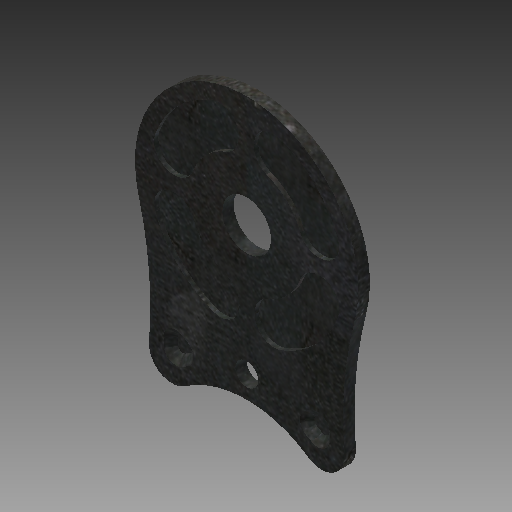
# Autodesk Inventor part: 201-09
Saved by Autodesk Inventor 2019 (Build 230136000, 136)
## iProperties
Company: Autodesk Inc.
Created: 2007-11-01
Part Number: 201-09
Document SubType Name: Modeling
Designer: Autodesk Inc.
Density: 7.85 g/cm^3
Mass: 170.342 g
Surface Area: 144.32 cm^2
Volume: 21.6997 cm^3
Material: Steel
Description: SIDE PIVOT PLATE
Appearance: Plate
Component Category: Lower Component
Author: Inventor
Autodesk Inventor part; units mm, degrees
ref_plane "YZ Plane" through (0, 0, 0) normal (1, 0, 0) x (0, 1, 0)
ref_plane "XZ Plane" through (0, 0, 0) normal (0, 1, 0) x (-1, 0, 0)
ref_plane "XY Plane" through (0, 0, 0) normal (0, 0, 1) x (1, 0, 0)
sketch "Sketch1" plane through (0, 0, 0) normal (0, 0, 1) x (1, 0, 0)
  arc A0 (37.7266, -9.8844) -> (-37.7266, -9.8844) centre (0, 0) ccw
  arc A1 (-34.0962, -52.1712) -> (-21.585, -59.437) centre (-26.125, -52.85) ccw
  arc A2 (21.585, -59.437) -> (34.0962, -52.1712) centre (26.125, -52.85) ccw
  arc A3 (-34.0962, -52.1712) -> (-37.7266, -9.8844) centre (-158.6454, -41.565) ccw
  line L0 (0, 64.9508) -> (0, -116.7047) projected
  arc A4 (21.585, -59.437) -> (-21.585, -59.437) centre (0, -90.7539) ccw
  arc A5 (37.7266, -9.8844) -> (34.0962, -52.1712) centre (158.6454, -41.565) ccw
  dimension "d0" = 16
  dimension "d2" = 78
  dimension "d3" = 52.85
  dimension "d5" = 26.125
  dimension "d8" = 317.2907
  dimension "d9" = 26.125
  dimension "d10" = 38.035
  constraints: 13 point on circle, 6 centre point, 4 tangent, 3 symmetric about line, 1 coincident, 1 point on line, 1 other
  measures "d0" diameter of A1
  measures "d2" diameter of A0
  measures "d3" vertical distance of A1.centre point (0, 0)
  measures "d5" horizontal distance of A1.centre point (0, 0)
  measures "d8" distance of A5.centre A3.centre
  measures "d9" distance from line of L0 A2.centre
  measures "d10" radius of A4
extrude "Extrusion1" add sketch "Sketch1" against normal blind 4
sketch "Sketch2" plane through (0, 0, -4) normal (0, 0, -1) x (-1, 0, 0)
  arc A0 (37.7266, -9.8844) -> (-37.7266, -9.8844) centre (0, 0) ccw projected
  arc A1 (-34.0962, -52.1712) -> (-21.585, -59.437) centre (-26.125, -52.85) ccw projected
  arc A2 (21.585, -59.437) -> (-21.585, -59.437) centre (0, -90.7539) ccw projected
  line L0 (-27.275, -50.4758) -> (-27.275, -48.2242)
  line L1 (-21.575, -51.5151) -> (-23.525, -52.6409)
  line L2 (-23.525, -46.0591) -> (-21.575, -47.1849)
  arc A3 (-23.525, -46.0591) -> (-27.275, -48.2242) centre (-24.775, -48.2242) ccw
  arc A4 (-27.275, -50.4758) -> (-23.525, -52.6409) centre (-24.775, -50.4758) ccw
  arc A5 (-21.575, -51.5151) -> (-21.575, -47.1849) centre (-22.825, -49.35) ccw
  line L3 (0, -116.7047) -> (0, 64.9508) projected
  point P0 (-27.275, 27.8761)
  point P1 (-32.4256, -57.7797)
  point P2 (-9.7764, -53.9968)
  dimension "d13" = 60
  dimension "d14" = 60
  dimension "d15" = 2.5
  dimension "d16" = 22.825
  dimension "d17" = 49.35
  dimension "d18" = 60
  dimension "d19" = 1.95
  constraints: 9 point on circle, 6 end point, 6 tangent, 3 centre point, 3 point on line, 2 equal radius
  measures "d13" angle of L1 L0
  measures "d14" angle of L1 L2
  measures "d15" radius of A3
  measures "d16" horizontal distance of A0.centre A5.centre
  measures "d17" vertical distance of A0.centre A5.centre
  measures "d18" angle of L3 L1
  measures "d19" horizontal distance of A3.centre A5.centre
extrude "Extrusion2" add sketch "Sketch2" along normal blind 2.5
chamfer "Chamfer1" distance 2.5 angle 45 6 edges at (22.55, -52.078, -4) (26.025, -52.6409, -4) (27.275, -49.35, -4) (26.025, -46.0591, -4) (22.55, -46.622, -4) (20.325, -49.35, -4)
mirror "Mirror1" about plane through (0, 0, 0) normal (1, 0, 0) of "Extrusion2", "Chamfer1"
sketch "Sketch3" plane through (0, 0, 0) normal (0, 0, 1) x (1, 0, 0)
  line L0 (-23.525, -46.0591) -> (-21.575, -47.1849) projected
  arc A0 (-21.575, -51.5151) -> (-21.575, -47.1849) centre (-22.825, -49.35) ccw projected
  line L1 (-21.575, -51.5151) -> (-23.525, -52.6409) projected
  arc A1 (-27.275, -50.4758) -> (-23.525, -52.6409) centre (-24.775, -50.4758) ccw projected
  line L2 (-27.275, -50.4758) -> (-27.275, -48.2242) projected
  arc A2 (-23.525, -46.0591) -> (-27.275, -48.2242) centre (-24.775, -48.2242) ccw projected
  line L3 (-22.65, -54.1564) -> (-20.7, -53.0306)
  arc A3 (-20.7, -53.0306) -> (-20.7, -45.6694) centre (-22.825, -49.35) ccw
  line L4 (-20.7, -45.6694) -> (-22.65, -44.5436)
  arc A4 (-22.65, -44.5436) -> (-29.025, -48.2242) centre (-24.775, -48.2242) ccw
  line L5 (-29.025, -48.2242) -> (-29.025, -50.4758)
  arc A5 (-29.025, -50.4758) -> (-22.65, -54.1564) centre (-24.775, -50.4758) ccw
  dimension "d30" = 1.75
  constraints: 6 end point, 6 point on circle, 3 centre point, 5 other
  measures "d30" distance between parallel lines of L3 L1
extrude "Extrusion3" cut sketch "Sketch3" against normal blind 2.5 contours L0 A0 L1 A1 L2 A2 | A5 L5 A4 L4 A3 L3
chamfer "Chamfer2" distance 2.5 angle 45 6 edges at (-26.9, -54.1564, -2.5) (-21.675, -53.5935, -2.5) (-18.575, -49.35, -2.5) (-21.675, -45.1065, -2.5) (-26.9, -44.5436, -2.5) (-29.025, -49.35, -2.5)
mirror "Mirror2" about plane through (0, 0, 0) normal (1, 0, 0) of "Extrusion3", "Chamfer2"
sketch "Sketch4" plane through (0, 0, 0) normal (0, 0, 1) x (1, 0, 0)
  circle A0 centre (0, 0) radius 8.5
  line L0 (0, 0) -> (0, -45)
  circle A1 centre (0, -45) radius 4
  dimension "d31" = 17
  dimension "d32" = 45
  dimension "d33" = 8
  constraints: 2 centre point, 2 coincident, 2 end point, 1 vertical
  measures "d31" diameter of A0
  measures "d32" distance of L0.start L0.end
  measures "d33" diameter of A1
extrude "Extrusion4" cut sketch "Sketch4" against normal through all
sketch "Sketch5" plane through (0, 0, 0) normal (0, 0, 1) x (1, 0, 0)
  circle A0 centre (0, 0) radius 8.5 projected
  line L0 (-29.025, -50.4758) -> (-29.025, -48.2242) projected
  arc A1 (37.7266, -9.8844) -> (-37.7266, -9.8844) centre (0, 0) ccw projected
  arc A2 (-2.8, 33.8845) -> (-33.908, 2.5) centre (0, 0) ccw
  arc A3 (-2.8, 19.803) -> (-19.8431, 2.5) centre (0, 0) ccw
  line L1 (-2.8, 33.8845) -> (-2.8, 19.803)
  line L2 (-19.8431, 2.5) -> (-33.908, 2.5)
  dimension "d36" = 68
  dimension "d37" = 40
  dimension "d38" = 2.5
  dimension "d39" = 2.8
  constraints: 4 end point, 4 point on circle, 2 centre point, 2 coincident, 1 parallel, 1 perpendicular
  measures "d36" diameter of A2
  measures "d37" diameter of A3
  measures "d38" distance from line of L2 A0.centre
  measures "d39" distance from line of A0.centre L1
extrude "Extrusion5" cut sketch "Sketch5" against normal blind 1.5 contours L1 A3 L2 A2
fillet "Fillet1" radius 6.75 4 edges at (-2.8, 33.8845, -0.75) (-2.8, 19.803, -0.75) (-19.8431, 2.5, -0.75) (-33.908, 2.5, -0.75)
pattern_circular "Circular Pattern1" count 4 over 360 about axis through (0, 0, 0) along (0, 0, -1) of "Extrusion5", "Fillet1"
body "Solid1"
